Axe 2 (Autodesk Fusion 360 design; units mm, degrees)
Autodesk Fusion 360 part; units mm, degrees
sketch "Sketch1" plane through (0, 0, 0) normal (0, 0, 1) x (1, 0, 0)
  circle A0 centre (0, 0) radius 20
  line L0 (4.0415, 0) -> (2.0207, 3.5)
  line L1 (2.0207, 3.5) -> (-2.0207, 3.5)
  line L2 (-2.0207, 3.5) -> (-4.0415, 0)
  line L3 (-4.0415, 0) -> (-2.0207, -3.5)
  line L4 (-2.0207, -3.5) -> (2.0207, -3.5)
  line L5 (2.0207, -3.5) -> (4.0415, 0)
  dimension "d1" = 40
  dimension "d10" = 7
  constraint coincident A0.centre origin
  constraint horizontal L1
  measures "d1" diameter of A0
  measures "d10" distance of L1 L4
extrude "Extrude1" add sketch "Sketch1" along normal blind 2
sketch "Sketch2" plane through (0, 0, 2) normal (0, 0, 1) x (-1, 0, 0)
  circle A0 centre (0, 0) radius 20
  circle A1 centre (0, 0) radius 8
  line L0 (-4.0415, 0) -> (-2.0207, 3.5)
  line L1 (-2.0207, 3.5) -> (2.0207, 3.5)
  line L2 (2.0207, 3.5) -> (4.0415, 0)
  line L3 (4.0415, 0) -> (2.0207, -3.5)
  line L4 (2.0207, -3.5) -> (-2.0207, -3.5)
  line L5 (-2.0207, -3.5) -> (-4.0415, 0)
  dimension "d4" = 16
  constraint concentric A0 A1
  measures "d4" diameter of A1
extrude "Extrude2" add sketch "Sketch2" along normal blind 0.3 contours A1
sketch "Sketch3" plane through (0, 0, 2.3) normal (0, 0, 1) x (-1, 0, 0)
  circle A0 centre (0, 0) radius 8
  circle A1 centre (0, 0) radius 6
  line L0 (2.0207, -3.5) -> (-2.0207, -3.5)
  line L1 (-2.0207, -3.5) -> (-4.0415, 0)
  line L2 (-4.0415, 0) -> (-2.0207, 3.5)
  line L3 (-2.0207, 3.5) -> (2.0207, 3.5)
  line L4 (2.0207, 3.5) -> (4.0415, 0)
  line L5 (4.0415, 0) -> (2.0207, -3.5)
  dimension "d7" = 12
  constraint coincident A0.centre A1.centre
  measures "d7" diameter of A1
extrude "Extrude3" add sketch "Sketch3" along normal blind 3.5 contours A1
named bodies: "Axe2"
